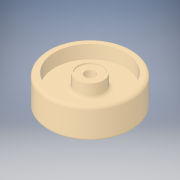
# Autodesk Inventor part: Wheel
Saved by Autodesk Inventor 2017 (Build 210142000, 142)
## iProperties
Created: 2016-06-14
Part Number: Wheel
Material: Polyethylene, High Density
Document SubType Name: Modeling
Designer: Dakota Marin
Density: 0.952 g/cm^3
Appearance: Smooth - Off-White
Author: Dakota Marin
Autodesk Inventor part; units mm, degrees
ref_plane "YZ Plane" through (0, 0, 0) normal (1, 0, 0) x (0, 1, 0)
ref_plane "XZ Plane" through (0, 0, 0) normal (0, 1, 0) x (-1, 0, 0)
ref_plane "XY Plane" through (0, 0, 0) normal (0, 0, 1) x (1, 0, 0)
sketch "Sketch1" plane through (0, 0, 0) normal (0, 0, 1) x (1, 0, 0)
  line L0 (0.0819, 48.1439) -> (0.0819, -16.0521)
  line L1 (0.0819, 0.0886) -> (20.0819, 0.0886)
  line L2 (20.0819, 0.0886) -> (20.0819, 20.0886)
  line L3 (20.0819, 20.0886) -> (0.0819, 20.0886)
  line L4 (0.0819, 20.0886) -> (0.0819, 0.0886)
  line L5 (0.0819, 0.0886) -> (62.5819, 0.0886)
  line L6 (62.5819, 0.0886) -> (62.5819, -4.9114)
  line L7 (62.5819, -4.9114) -> (0.0819, -4.9114)
  line L8 (0.0819, -4.9114) -> (0.0819, 0.0886)
  line L9 (62.5819, 0.0886) -> (52.5819, 0.0886)
  line L10 (52.5819, 0.0886) -> (52.5819, 20.0886)
  line L11 (52.5819, 20.0886) -> (62.5819, 20.0886)
  line L12 (62.5819, 20.0886) -> (62.5819, 0.0886)
  line L13 (0.0819, -4.9114) -> (20.0819, -4.9114)
  line L14 (20.0819, -4.9114) -> (20.0819, -24.9114)
  line L15 (20.0819, -24.9114) -> (0.0819, -24.9114)
  line L16 (0.0819, -24.9114) -> (0.0819, -4.9114)
  line L17 (52.5819, -4.9114) -> (62.5819, -4.9114)
  line L18 (62.5819, -4.9114) -> (62.5819, -24.9114)
  line L19 (62.5819, -24.9114) -> (52.5819, -24.9114)
  line L20 (52.5819, -24.9114) -> (52.5819, -4.9114)
  dimension "d4" = 62.5
  dimension "d5" = 20
  dimension "d6" = 20
  dimension "d7" = 20
  dimension "d8" = 10
  dimension "d10" = 20
  dimension "d11" = 20
  dimension "d12" = 5
  dimension "d13" = 20
  dimension "d14" = 10
  constraints: 42 end point, 10 parallel, 5 horizontal, 5 perpendicular, 2 point on line, 2 vertical
  measures "d4" distance of L6.end L7.end
  measures "d5" distance of L1.end L2.end
  measures "d6" distance of L11.end L5.end
  measures "d7" distance of L2.end L3.end
  measures "d8" distance of L10.end L11.end
  measures "d10" distance of L17.end L18.end
  measures "d11" distance of L13.end L14.end
  measures "d12" distance of L5.end L6.end
  measures "d13" distance of L14.end L15.end
  measures "d14" distance of L18.end L19.end
revolve "Revolution2" add sketch "Sketch1" angle 360 about axis through (0.0819, 48.1439, 0) along (0, -1, 0)
fillet "Fillet1" radius 5 2 edges at (-62.4181, 20.0886, 0) (-62.4181, -24.9114, 0)
fillet "Fillet2" radius 5 1 edges at (-19.9181, 0.0886, 0)
fillet "Fillet3" radius 5 1 edges at (-19.9181, -4.9114, 0)
sketch "Sketch2" plane through (0.0819, 20.0886, 0) normal (0, 1, 0) x (1, 0, 0)
  circle A0 centre (-0.0819, 0) radius 18
  dimension "d21" = 36
  constraints: 1 centre point, 1 coincident
  measures "d21" diameter of A0
extrude "Extrusion1" cut sketch "Sketch2" against normal blind 2
sketch "Sketch3" plane through (0.0819, -24.9114, 0) normal (0, -1, 0) x (1, 0, 0)
  circle A0 centre (-0.0819, 0) radius 18
  dimension "d22" = 36
  constraints: 1 centre point, 1 coincident
  measures "d22" diameter of A0
extrude "Extrusion2" cut sketch "Sketch3" against normal blind 2
sketch "Sketch4" plane through (0, 18.0886, 0) normal (0, 1, 0) x (1, 0, 0)
  circle A0 centre (0, 0) radius 7.5
  dimension "d25" = 15
  constraints: 1 centre point, 1 coincident
  measures "d25" diameter of A0
extrude "Extrusion3" cut sketch "Sketch4" against normal through all
body "Solid2"
